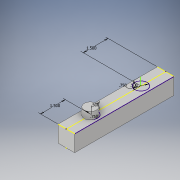
# Autodesk Inventor part: Lego
Saved by Autodesk Inventor 2017 (Build 210142000, 142)
## iProperties
Created: 2017-10-26
Part Number: Lego
Material: Generic
Document SubType Name: Modeling
Designer: Aidan_Moga
Density: 1 g/cm^3
Appearance: Default
Author: Aidan_Moga
Autodesk Inventor part; units mm, degrees
ref_plane "YZ Plane" through (0, 0, 0) normal (1, 0, 0) x (0, 1, 0)
ref_plane "XZ Plane" through (0, 0, 0) normal (0, 1, 0) x (-1, 0, 0)
sketch "Sketch1" plane through (0, 0, 0) normal (0, 1, 0) x (-1, 0, 0)
  line L0 (0, 0) -> (25.4, 0)
  line L1 (25.4, 0) -> (25.4, -152.4)
  line L2 (25.4, -152.4) -> (0, -152.4)
  line L3 (0, -152.4) -> (0, 0)
  dimension "d0" = 25.4
  dimension "d2" = 152.4
  constraints: 8 end point, 2 parallel, 1 horizontal, 1 perpendicular
  measures "d0" distance of L1.end L2.end
  measures "d2" distance of L0.end L1.end
extrude "Extrusion1" add sketch "Sketch1" along normal blind 25.4
sketch "Sketch2" plane through (0, 25.4, 0) normal (0, 1, 0) x (1, 0, 0)
  circle A0 centre (-12.7, 38.1) radius 9.525
  circle A1 centre (-12.7, 114.3) radius 9.525
  line L0 (0, 0) -> (0, 152.4) projected
  line L1 (0, 0) -> (0, 152.4)
  line L2 (-25.4, 0) -> (0, 0) projected
  line L3 (0, 152.4) -> (-25.4, 152.4) projected
  point P0 (-12.7, 0)
  point P1 (-12.7, 152.4)
  dimension "d5" = 19.05
  dimension "d6" = 19.05
  dimension "d7" = 38.1
  dimension "d8" = 38.1
  constraints: 2 centre point, 2 end point, 2 midpoint, 2 vertical alignment, 1 collinear
  measures "d5" diameter of A0
  measures "d6" diameter of A1
  measures "d7" distance from line of A0.centre L2
  measures "d8" distance from line of A1.centre L3
ref_plane "Work Plane2" through (-12.7, 25.4, 0) normal (1, 0, 0) x (0, 0, -1)
sketch "Sketch3" plane through (-12.7, 25.4, 0) normal (1, 0, 0) x (0, 0, -1)
  line L0 (0, 0) -> (152.4, 0) projected
  line L1 (37.8661, 0) -> (50.5661, 0)
  line L2 (113.6104, 0) -> (113.6104, 12.7)
  point P0 (0, -25.4)
  dimension "d11" = 12.7
  dimension "d12" = 12.7
  constraints: 4 end point, 3 point on line, 1 vertical
  measures "d11" distance of L1.start L1.end
  measures "d12" distance of L2.start L2.end
sketch "Sketch4" plane through (-12.7, 25.4, 0) normal (1, 0, 0) x (0, 0, -1)
  line L0 (27.5288, 0.0165) -> (36.6748, 0.0165)
  line L1 (36.6748, 0.0165) -> (36.6748, 11.0679)
  line L2 (36.6748, 11.0679) -> (27.5288, 11.0679)
  line L3 (27.5288, 11.0679) -> (27.5288, 0.0165)
  point P0 (0, -25.4)
  constraints: 8 end point, 2 parallel, 1 horizontal, 1 perpendicular
revolve "Revolution1" add sketch "Sketch4" angle 360 about axis through (-12.7, 25.4165, -36.6748) along (0, -1, 0)
body "Solid1"
